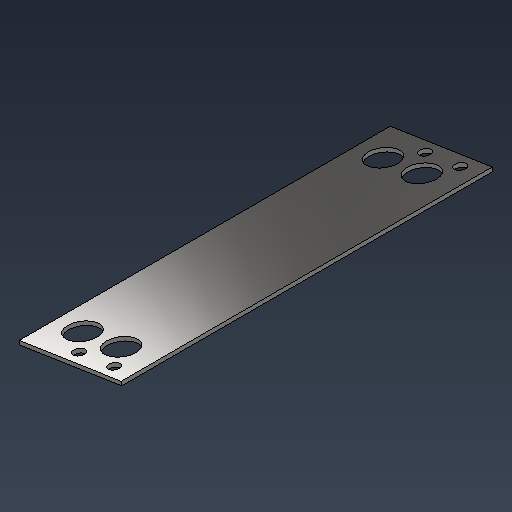
# Autodesk Inventor part: SteelFront
Saved by Autodesk Inventor 2026.2 (Build 302298010, 298A)
## iProperties
Created: 2026-04-07
Part Number: SteelFront
Material: Steel, Alloy
Document SubType Name: Modeling
Designer: szymo
Density: 7.73 g/cm^3
Appearance: Semi-Polished(2)
Mass: 19.6905 g
Surface Area: 54.8833 cm^2
Volume: 2.54729 cm^3
Author: szymo
Autodesk Inventor part; units mm, degrees
ref_plane "YZ Plane" through (0, 0, 0) normal (1, 0, 0) x (0, 1, 0)
ref_plane "XZ Plane" through (0, 0, 0) normal (0, 1, 0) x (-1, 0, 0)
ref_plane "XY Plane" through (0, 0, 0) normal (0, 0, 1) x (1, 0, 0)
sketch "Sketch1" plane through (0, 0, 0) normal (0, 0, 1) x (1, 0, 0)
  line L0 (0.65, -95.0088) -> (0.65, -82.5008) construction
  line L1 (2.65, -82.5008) -> (2.65, -91.0088) construction
  line L2 (2.65, -91.0088) -> (4.65, -91.0088) construction
  line L3 (4.65, -91.0088) -> (0.65, -95.0088) construction
  circle A0 centre (15.35, -55.1458) radius 14.7 construction
  line L4 (3.0006, -90.8088) -> (30.45, -86.6259)
  line L5 (30.45, -86.6259) -> (30.2994, -85.6374)
  line L6 (30.2994, -85.6374) -> (2.85, -89.8202)
  line L7 (2.85, -89.8202) -> (3.0006, -90.8088)
  line L8 (30.45, -86.6259) -> (30.45, -70.1877) construction
  line L9 (25.65, -86.3458) -> (5.15, -86.3458) projected
  line L10 (5.15, -86.3458) -> (5.15, -69.8458) projected
  line L11 (25.65, -69.8458) -> (5.15, -69.8458) projected
  line L12 (25.65, -86.3458) -> (25.65, -69.8458) projected
  line L13 (0.65, -82.5008) -> (2.65, -82.5008) projected
  dimension "d0" = 1
  dimension "d1" = 0.2
  dimension "d2" = 0.2
  dimension "d3" = 0.4
  dimension "d4" = 0
  constraints: 10 end point, 2 parallel, 1 perpendicular, 1 vertical
  measures "d0" distance between parallel lines of L6 L4
  measures "d1" distance from line of L1 L6.end
  measures "d2" distance from line of L2 L4.start
  measures "d3" distance edge to line of A0 L8
  measures "d4" distance from line of L6 L9.start
extrude "Extrusion1" add sketch "Sketch1" along normal mid plane 100 contours L7 L6 L5 L4
sketch "Sketch2" plane through (30.45, -86.6259, -50) normal (0.1506443, -0.988588, 0) x (0.988588, 0.1506443, 0)
  line L0 (-25.9454, 16.5) -> (-25.9454, 84.5) projected
  line L1 (-27.9685, 0) -> (-27.9685, 1) projected
  circle A0 centre (-5.2783, 96.6469) radius 1.5
  circle A1 centre (-14.8697, 96.6469) radius 1.5
  circle A2 centre (-14.8697, 3.3531) radius 1.5
  circle A3 centre (-5.2783, 3.3531) radius 1.5
  circle A4 centre (-9.5918, 90.5) radius 4
  circle A5 centre (-20.1476, 90.5) radius 4
  circle A6 centre (-9.5918, 9.5) radius 4
  circle A7 centre (-20.1476, 9.5) radius 4
  line L2 (-27.9685, 17.5) -> (-27.3313, 17.5) projected
  line L3 (-27.3313, 17.5) -> (-27.3313, 1) projected
  line L4 (-2.2753, 15.5) -> (-24.9339, 15.5) projected
  line L5 (-13.8886, 7.2533) -> (-16.5988, 7.2533) projected
  line L6 (-27.3313, 1) -> (-27.9685, 1) projected
  line L7 (-27.9685, 17.5) -> (-27.9685, 82.5) projected
  line L8 (-2.2753, 84.5) -> (-25.9454, 84.5) projected
  ellipse E0 centre (-9.963, 9.5) end of major axis (-5.4324, 9.5) minor radius 4.5 (-13.8886, 7.2533) -> (-13.8886, 11.7467) ccw projected
  circle A8 centre (-15.2437, 96.3698) radius 2.25 projected
  circle A9 centre (-5.2753, 96.3698) radius 2.25 projected
  line L9 (-27.3313, 82.5) -> (-27.9685, 82.5) projected
  line L10 (-2.2753, 0) -> (-27.9685, 0) projected
  line L11 (-2.2753, 15.5) -> (-2.2753, 0) projected
  ellipse E1 centre (-24.9339, 16.5) end of major axis (-25.9454, 16.5) minor radius 1 (-25.9454, 16.5) -> (-24.9339, 15.5) ccw projected
  line L12 (-2.2753, 84.5) -> (-2.2753, 100) projected
  line L13 (-2.2753, 100) -> (-27.9685, 100) projected
  line L14 (-27.9685, 99) -> (-27.9685, 100) projected
  line L15 (-27.9685, 99) -> (-27.3313, 99) projected
  line L16 (-27.3313, 99) -> (-27.3313, 82.5) projected
  ellipse E2 centre (-20.5244, 90.5) end of major axis (-15.9938, 90.5) minor radius 4.5 (-16.5988, 92.7467) -> (-16.5988, 88.2533) ccw projected
  line L17 (-16.5988, 92.7467) -> (-13.8886, 92.7467) projected
  ellipse E3 centre (-9.963, 90.5) end of major axis (-5.4324, 90.5) minor radius 4.5 (-13.8886, 88.2533) -> (-13.8886, 92.7467) ccw projected
  line L18 (-13.8886, 88.2533) -> (-16.5988, 88.2533) projected
  circle A10 centre (-15.2437, 3.6302) radius 2.25 projected
  circle A11 centre (-5.2753, 3.6302) radius 2.25 projected
  ellipse E4 centre (-20.5244, 9.5) end of major axis (-15.9938, 9.5) minor radius 4.5 (-16.5988, 11.7467) -> (-16.5988, 7.2533) ccw projected
  line L19 (-16.5988, 11.7467) -> (-13.8886, 11.7467) projected
  point P0 (-17.0528, 50)
  point P1 (-28.5444, 1)
  point P2 (-16.268, 7.2533)
  point P3 (-16.3079, 7.2533)
  point P4 (-16.3688, 7.2533)
  point P5 (-16.5217, 7.2533)
  point P6 (-16.5463, 7.2533)
  point P7 (-14.6243, 7.2533)
  point P8 (-17.1998, 7.2533)
  point P9 (-9.892, 13.95)
  point P10 (-28.626, 82.5)
  point P11 (-14.5461, 11.7467)
  dimension "d7" = 3
  dimension "d8" = 3
  dimension "d9" = 3
  dimension "d10" = 3
  dimension "d13" = 8
  dimension "d14" = 8
  dimension "d15" = 8
  dimension "d16" = 8
  constraints: 8 centre point, 8 other
  measures "d7" diameter of A0
  measures "d8" diameter of A1
  measures "d9" diameter of A2
  measures "d10" diameter of A3
  measures "d13" diameter of A4
  measures "d14" diameter of A5
  measures "d15" diameter of A7
  measures "d16" diameter of A6
extrude "Extrusion2" cut sketch "Sketch2" against normal through all contours A0 | A1 | A2 | A3 | A4 | A5 | A6 | A7
equation "\"d14\" = d13"
equation "\"d15\" = d13"
equation "\"d16\" = d13"
body "Solid1"
